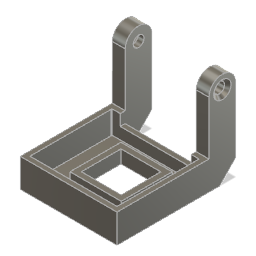
Pi case for camera top v3 (Autodesk Fusion 360 design; units mm, degrees)
Autodesk Fusion 360 part; units mm, degrees
sketch "Sketch1" plane through (0, 0, 0) normal (0, 1, 0) x (1, 0, 0)
  line L0 (0, 0) -> (29.58, 0)
  line L1 (29.58, 0) -> (29.58, -28.08)
  line L2 (0, 0) -> (29.58, 0)
  line L3 (29.58, 0) -> (29.58, -28.08)
  line L4 (29.58, -28.08) -> (0, -28.08)
  line L5 (0, -28.08) -> (0, 0)
  dimension "d1" = 29.58
  dimension "d2" = 28.08
extrude "Extrude1" add sketch "Sketch1" along normal blind 8.83
sketch "Sketch2" plane through (0, 8.83, 0) normal (0, 1, 0) x (-1, 0, 0)
  line L0 (0, 28.08) -> (-29.58, 28.08)
  line L1 (-29.58, 28.08) -> (-29.58, 0)
  line L2 (-29.58, 0) -> (0, 0)
  line L3 (0, 0) -> (0, 28.08)
  line L4 (-29.58, 14.04) -> (-22.61, 14.04)
  line L5 (-14.79, 28.08) -> (-14.79, 19.82)
  line L6 (0, 14.04) -> (-6.97, 14.04)
  line L7 (-14.79, 0) -> (-14.79, 4.24)
  line L8 (-6.97, 14.04) -> (-14.79, 14.04)
  line L9 (-14.79, 14.04) -> (-14.79, 19.82)
  line L10 (-14.79, 19.82) -> (-6.97, 19.82)
  line L11 (-6.97, 19.82) -> (-6.97, 14.04)
  line L12 (-14.79, 19.82) -> (-22.61, 19.82)
  line L13 (-22.61, 19.82) -> (-22.61, 14.04)
  line L14 (-22.61, 14.04) -> (-14.79, 14.04)
  line L15 (-14.79, 14.04) -> (-14.79, 19.82)
  line L16 (-22.61, 14.04) -> (-14.79, 14.04)
  line L17 (-14.79, 14.04) -> (-14.79, 4.24)
  line L18 (-14.79, 4.24) -> (-22.61, 4.24)
  line L19 (-22.61, 4.24) -> (-22.61, 14.04)
  line L20 (-14.79, 4.24) -> (-6.97, 4.24)
  line L21 (-6.97, 4.24) -> (-6.97, 14.04)
  line L22 (-6.97, 14.04) -> (-14.79, 14.04)
  line L23 (-14.79, 14.04) -> (-14.79, 4.24)
  line L24 (-6.97, 4.24) -> (-8.71, 4.24)
  line L25 (-8.71, 4.24) -> (-8.71, 5.98)
  line L26 (-8.71, 5.98) -> (-6.97, 5.98)
  line L27 (-6.97, 5.98) -> (-6.97, 4.24)
  line L28 (-22.61, 19.82) -> (-20.87, 19.82)
  line L29 (-20.87, 19.82) -> (-20.87, 18.08)
  line L30 (-20.87, 18.08) -> (-22.61, 18.08)
  line L31 (-22.61, 18.08) -> (-22.61, 19.82)
  line L32 (-8.71, 5.98) -> (-20.87, 5.98)
  line L33 (-20.87, 5.98) -> (-20.87, 18.08)
  line L34 (-20.87, 18.08) -> (-8.71, 18.08)
  line L35 (-8.71, 18.08) -> (-8.71, 5.98)
  line L36 (0, 28.08) -> (-1.8, 28.08)
  line L37 (-1.8, 28.08) -> (-1.8, 26.28)
  line L38 (-1.8, 26.28) -> (0, 26.28)
  line L39 (0, 26.28) -> (0, 28.08)
  line L40 (-29.58, 0) -> (-27.78, 0)
  line L41 (-27.78, 0) -> (-27.78, 1.8)
  line L42 (-27.78, 1.8) -> (-29.58, 1.8)
  line L43 (-29.58, 1.8) -> (-29.58, 0)
  line L44 (-1.8, 26.28) -> (-27.78, 26.28)
  line L45 (-27.78, 26.28) -> (-27.78, 1.8)
  line L46 (-27.78, 1.8) -> (-1.8, 1.8)
  line L47 (-1.8, 1.8) -> (-1.8, 26.28)
  dimension "d5" = 6.97
  dimension "d6" = 8.26
  dimension "d7" = 6.97
  dimension "d8" = 4.24
  dimension "d9" = 1.74
  dimension "d10" = 1.74
  dimension "d11" = 1.74
  dimension "d12" = 1.74
  dimension "d13" = 1.8
  dimension "d14" = 1.8
  dimension "d15" = 1.8
  dimension "d16" = 1.8
  measures "d14" distance of L2.end
  measures "d16" distance of L2.end
extrude "Extrude3" cut sketch "Sketch2" against normal blind 17 contours L8 L9 L15 L22 L34 L35 | L9 L14 L15 L16 L33 L34 | L8 L17 L22 L23 L32 L35 | L14 L16 L17 L23 L32 L33
extrude "Extrude2" cut sketch "Sketch2" against normal blind 7 contours L5 L6 L10 L11 L44 L47 | L4 L5 L12 L13 L28 L31 L44 L45 | L6 L7 L20 L21 L24 L27 L46 L47 | L4 L7 L18 L19 L45 L46
extrude "Extrude4" cut sketch "Sketch2" against normal blind 4.75 contours L8 L9 L10 L11 L15 L22 L34 L35 | L9 L12 L15 L29 L34 | L8 L21 L22 L26 L35 | L12 L13 L28 L29 L30 L31 | L20 L21 L24 L25 L26 L27 | L13 L14 L16 L30 L33 | L14 L16 L17 L18 L19 L23 L32 L33 | L17 L20 L23 L25 L32
sketch "Sketch3" plane through (29.58, 0, 0) normal (1, 0, 0) x (0, 0, -1)
  line L0 (-28.08, 0) -> (0, 0)
  line L1 (0, 0) -> (0, 8.83)
  line L2 (0, 8.83) -> (-28.08, 8.83)
  line L3 (-28.08, 8.83) -> (-28.08, 0)
  line L4 (0, 0) -> (3.32, 0)
  line L5 (3.32, 0) -> (8.22, 5.12)
  line L6 (8.22, 5.12) -> (8.22, 25.12)
  line L7 (8.22, 25.12) -> (4.12, 25.12)
  circle A0 centre (4.12, 25.12) radius 4.1
  line L8 (0.0202, 25.1643) -> (0, 8.83)
  circle A1 centre (4.12, 25.12) radius 1.65
  dimension "d23" = 3.32
  dimension "d26" = 20
  dimension "d27" = 4.1
  dimension "d28" = 3.3
  measures "d23" distance of L0.end
  measures "d28" diameter of A1
extrude "Extrude5" add sketch "Sketch3" against normal up to surface (29.58 mm away) contours L1 L4 L5 L6 A0 L8 | A0
chamfer "Chamfer1" distance 1 angle 45 1 edges at (29.58, 25.7167, -2.5817)
sketch "Sketch4" plane through (0, 0, 0) normal (-1, 0, 0) x (0, 0, 1)
  circle A0 centre (-4.12, 25.12) radius 1.65
  line L0 (-3.32, 0) -> (28.08, 0)
  line L1 (28.08, 0) -> (28.08, 8.83)
  line L2 (28.08, 8.83) -> (0, 8.83)
  line L3 (0, 8.83) -> (-0.0202, 25.1643)
  arc A1 (-0.0202, 25.1643) -> (-8.22, 25.12) centre (-4.12, 25.12) ccw
  line L4 (-8.22, 25.12) -> (-8.22, 5.12)
  line L5 (-8.22, 5.12) -> (-3.32, 0)
  line L6 (-4.12, 25.12) -> (-4.12, 26.77)
  line L7 (-4.12, 25.12) -> (-2.47, 25.12) construction
  line L8 (-5.5489, 25.945) -> (-7.4542, 27.045)
  line L9 (-5.5489, 24.295) -> (-7.4542, 23.195)
  line L10 (-4.12, 23.47) -> (-4.12, 21.27)
  line L11 (-2.6911, 24.295) -> (-0.7858, 23.195)
  line L12 (-2.6911, 25.945) -> (-0.7858, 27.045)
  line L13 (-4.12, 28.97) -> (-0.7858, 27.045)
  line L14 (-0.7858, 27.045) -> (-0.7858, 23.195)
  line L15 (-0.7858, 23.195) -> (-4.12, 21.27)
  line L16 (-4.12, 21.27) -> (-7.4542, 23.195)
  line L17 (-7.4542, 23.195) -> (-7.4542, 27.045)
  circle A2 centre (-4.12, 25.12) radius 1.65
  line L18 (-4.12, 28.97) -> (-7.4542, 27.045)
  dimension "d32" = 2.2
extrude "Extrude6" cut sketch "Sketch4" against normal blind 2.2 contours A0 L11 L12 L14 A2 | A0 L8 L12 L13 A2 L18 | A0 L10 L11 L15 A2 | A0 L9 L10 L16 A2 | A0 L8 L9 L17 A2
sketch "Sketch5" plane through (0, 0, -8.22) normal (0, 0, -1) x (-1, 0, 0)
  line L0 (0, 5.12) -> (0, 25.12)
  line L1 (0, 25.12) -> (-29.58, 25.12)
  line L2 (-29.58, 25.12) -> (-29.58, 5.12)
  line L3 (-29.58, 5.12) -> (0, 5.12)
  line L4 (0, 0) -> (-3.96, 0)
  line L5 (-29.58, 0) -> (0, 0)
  line L6 (-29.58, 0) -> (-25.62, 0)
  line L7 (-25.62, 0) -> (-4, 0)
  line L8 (-4, 0) -> (-4, 29)
  line L9 (-4, 29) -> (-25.62, 29)
  line L10 (-25.62, 29) -> (-25.62, 0)
  line L11 (-25.62, 29) -> (-4, 29)
  line L12 (-4, 29) -> (-4, 33)
  line L13 (-4, 33) -> (-25.62, 33)
  line L14 (-25.62, 33) -> (-25.62, 29)
  dimension "d39" = 3.96
  dimension "d40" = 3.96
  measures "d39" distance of L4.start
extrude "Extrude8" cut sketch "Sketch5" against normal blind 8.24 contours L3 L5 L7 L8 L10 | L1 L3 L8 L10 | L1 L8 L9 L10 L11 | L9 L11 L12 L13 L14
extrude "Extrude7" cut sketch "Sketch5" against normal blind 8.24 contours L3 L5 L7 L8 L10 | L1 L3 L8 L10 | L1 L8 L9 L10 L11
chamfer "Chamfer2" distance 2 angle 45 1 edges at (14.81, 0, 0.02)
sketch "Sketch6" plane through (0, 0, 0.02) normal (0, 0, -1) x (-1, 0, 0)
  line L0 (-25.62, 2) -> (-4, 2)
  line L1 (-4, 2) -> (-4, 8.83)
  line L2 (-4, 8.83) -> (-25.62, 8.83)
  line L3 (-25.62, 8.83) -> (-25.62, 2)
  line L4 (-4, 8.83) -> (-25.62, 8.83)
  line L5 (-25.62, 8.83) -> (-25.62, 5.415)
  line L6 (-25.62, 5.415) -> (-4, 5.415)
  line L7 (-4, 5.415) -> (-4, 8.83)
extrude "Extrude9" cut sketch "Sketch6" against normal blind 8 contours L1 L2 L3 L4 L5 L6 L7
sketch "Sketch7" plane through (0, 8.83, 0) normal (0, 1, 0) x (-1, 0, 0)
  line L0 (-25.62, 0) -> (-25.62, 1.8)
  line L1 (-25.62, 1.8) -> (-27.78, 1.8)
  line L2 (-27.78, 1.8) -> (-27.78, 26.28)
  line L3 (-27.78, 26.28) -> (-1.8, 26.28)
  line L4 (-1.8, 26.28) -> (-1.8, 1.8)
  line L5 (-1.8, 1.8) -> (-4, 1.8)
  line L6 (-4, 1.8) -> (-4, 0)
  line L7 (-4, 0) -> (0, 0)
  line L8 (0, 0) -> (0, 28.08)
  line L9 (0, 28.08) -> (-29.58, 28.08)
  line L10 (-29.58, 28.08) -> (-29.58, 0)
  line L11 (-29.58, 0) -> (-25.62, 0)
  line L12 (-1.8, 1.8) -> (-1.5, 1.8)
  line L13 (-1.5, 1.8) -> (-1.5, 1.5)
  line L14 (-1.5, 1.5) -> (-1.8, 1.5)
  line L15 (-1.8, 1.5) -> (-1.8, 1.8)
  line L16 (-1.8, 1.5) -> (-4, 1.5)
  line L17 (-1.8, 26.28) -> (-1.5, 26.28)
  line L18 (-1.5, 26.28) -> (-1.5, 26.58)
  line L19 (-1.5, 26.58) -> (-1.8, 26.58)
  line L20 (-1.8, 26.58) -> (-1.8, 26.28)
  line L21 (-1.5, 1.8) -> (-1.5, 26.28)
  line L22 (-27.78, 26.28) -> (-28.08, 26.28)
  line L23 (-28.08, 26.28) -> (-28.08, 26.58)
  line L24 (-28.08, 26.58) -> (-27.78, 26.58)
  line L25 (-27.78, 26.58) -> (-27.78, 26.28)
  line L26 (-1.8, 26.58) -> (-27.78, 26.58)
  line L27 (-27.78, 1.8) -> (-28.08, 1.8)
  line L28 (-28.08, 1.8) -> (-28.08, 1.5)
  line L29 (-28.08, 1.5) -> (-27.78, 1.5)
  line L30 (-27.78, 1.5) -> (-27.78, 1.8)
  line L31 (-28.08, 26.58) -> (-28.08, 1.5)
  line L32 (-27.78, 1.5) -> (-25.62, 1.5014)
  dimension "d48" = 0.3
  dimension "d49" = 0.3
  dimension "d50" = 0.3
  dimension "d51" = 0.3
  dimension "d52" = 0.3
  dimension "d53" = 0.3
extrude "Extrude10" cut sketch "Sketch7" against normal up to surface (7 mm away) contours L0 L1 L30 L32 | L27 L28 L29 L30 L31 | L2 L22 L27 L31 | L3 L20 L25 L26 | L22 L23 L24 L25 L31 | L4 L12 L17 L21 | L17 L18 L19 L20 | L5 L6 L15 L16 | L12 L13 L14 L15
sketch "Sketch8" plane through (0, 5.415, 0) normal (0, 1, 0) x (-1, 0, 0)
  line L0 (-4, 1.8) -> (-25.62, 1.8)
  line L1 (-25.62, 1.8) -> (-25.62, 1.5014)
  line L2 (-25.62, 1.5014) -> (-25.62, 0.02)
  line L3 (-25.62, 0.02) -> (-4, 0.02)
  line L4 (-4, 0.02) -> (-4, 1.5)
  line L5 (-4, 1.5) -> (-4, 1.8)
  line L6 (-4, 1.5) -> (-25.62, 1.5)
  line L7 (-25.62, 1.5) -> (-25.62, 1.8)
  line L8 (-25.62, 1.8) -> (-4, 1.8)
  line L9 (-4, 1.8) -> (-4, 1.5)
extrude "Extrude11" cut sketch "Sketch8" against normal up to surface (3.585 mm away) contours L0 L1 L2 L5 L6 L7 L8 L9
